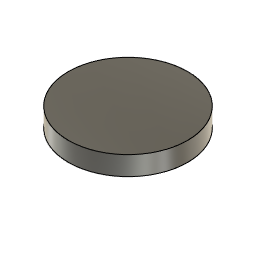
UNION SERVO-PIEZA v1 (Autodesk Fusion 360 design; units mm, degrees)
Autodesk Fusion 360 part; units mm, degrees
cylinder "CilindroPrimitivo1" add diameter 10 height 4 placed x (1, 0, 0) y (0, 1, 0) z (0, 0, 1) at (0, 0, 0)
sketch "Boceto2" plane through (0, 0, 4) normal (0, 0, 1) x (-1, 0, 0)
  circle A0 centre (0, 0) radius 5
  circle A1 centre (0, 0) radius 12.5
  constraint coincident A0.centre A1.centre
extrude "Extruir1" add sketch "Boceto2" along normal blind 4 contours A0 | A1
